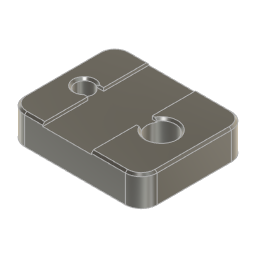
[a]_z_belt_clip_lower_x4 (Autodesk Fusion 360 design; units mm, degrees)
Autodesk Fusion 360 part; units mm, degrees
sketch "Sketch1" plane through (0, 0, 0) normal (0, 0, 1) x (1, 0, 0) in component "Component"
  line L0 (12.5, -10) -> (-12.5, -10)
  line L1 (-12.5, -10) -> (-12.5, 10)
  line L2 (-12.5, 10) -> (12.5, 10)
  line L3 (12.5, 10) -> (12.5, -10)
  line L4 (12.5, -10) -> (-12.5, 10) construction
  line L5 (-12.5, -10) -> (12.5, 10) construction
  line L6 (-12.5, 0) -> (12.5, 0) construction
  line L7 (0, 10) -> (0, -10) construction
  circle A0 centre (-8.25, 0) radius 1.7
  circle A1 centre (6.25, 0) radius 2.7
  dimension "d7" = 25
  dimension "d8" = 20
  dimension "d9" = 3.4
  dimension "d10" = 5.4
  dimension "d11" = 4.25
  dimension "d12" = 6.25
  constraint horizontal L0
  constraint perpendicular L0 L1
  constraint parallel L0 L2
  constraint parallel L1 L3
  constraint coincident L4 origin
  constraint coincident L5 origin
  constraint midpoint L1 L6.start
  constraint midpoint L3 L6.end
  constraint midpoint L2 L7.start
  constraint midpoint L0 L7.end
  constraint coincident L6 A0.centre
  constraint coincident L6 A1.centre
  measures "d7" distance of L1.end L2.end
  measures "d8" distance of L0.end L1.end
  measures "d9" diameter of A0
  measures "d10" diameter of A1
  measures "d11" distance of L1 A0.centre
  measures "d12" distance of L3 A1.centre
extrude "Extrude1" add sketch "Sketch1" along normal mid plane 5.6 in component "Component"
fillet "Fillet1" radius 3 4 edges at (-12.5, -10, 0) (12.5, -10, 0) (12.5, 10, 0) (-12.5, 10, 0) in component "Component"
chamfer "Chamfer1" distance 0.4 angle 45 12 edges at (0, -10, 2.8) (11.6213, -9.1213, 2.8) (12.5, 0, 2.8) (11.6213, 9.1213, 2.8) (0, 10, 2.8) (-11.6213, 9.1213, 2.8) (-12.5, 0, 2.8) (-11.6213, -9.1213, 2.8) (3.7327, 0.9764, 2.8) (-9.835, 0.6147, 2.8) (3.7327, -0.9764, -2.8) (-9.835, -0.6147, -2.8) in component "Component"
sketch "Sketch2" plane through (0, 0, 2.8) normal (0, 0, 1) x (-1, 0, 0) in component "Component"
  circle A0 centre (-6.25, 0) radius 3.1
  line L0 (9.5, 9.6) -> (-9.5, 9.6)
  arc A1 (-9.5, 9.6) -> (-12.1, 7) centre (-9.5, 7) ccw
  line L1 (-12.1, 7) -> (-12.1, -7)
  arc A2 (-12.1, -7) -> (-9.5, -9.6) centre (-9.5, -7) ccw
  line L2 (-9.5, -9.6) -> (9.5, -9.6)
  arc A3 (9.5, -9.6) -> (12.1, -7) centre (9.5, -7) ccw
  line L3 (12.1, -7) -> (12.1, 7)
  arc A4 (12.1, 7) -> (9.5, 9.6) centre (9.5, 7) ccw
  circle A5 centre (8.25, 0) radius 2.1
  line L4 (12.5, -10) -> (-12.5, -10)
  line L5 (12.5, 10) -> (12.5, -10)
  line L6 (-12.5, 10) -> (12.5, 10)
  line L7 (-12.5, -10) -> (-12.5, 10)
  line L8 (6.1, -10) -> (-3.1, -10)
  line L9 (-3.1, -10) -> (-3.1, 10)
  line L10 (-3.1, 10) -> (6.1, 10)
  line L11 (6.1, 10) -> (6.1, -10)
  dimension "d18" = 6.4
  dimension "d19" = 9.4
  constraint horizontal L8
  constraint vertical L9
  constraint horizontal L10
  constraint vertical L11
  constraint coincident L6 L9.end
  constraint coincident L4 L8.start
  measures "d18" distance of L5 L11
  measures "d19" distance of L7 L9
extrude "Extrude2" cut sketch "Sketch2" against normal blind 0.6 contours L0 L2 L9 L11 | L0 L6 L9 L10 L11 | L2 L4 L8 L9 L11 in component "Component"
sketch "Sketch3" plane through (0, 0, 2.8) normal (0, 0, 1) x (-1, 0, 0) in component "Component"
  line L0 (-3.1, -9.6) -> (-3.1, 9.6)
  line L1 (-3.1, 9.6) -> (-9.5, 9.6)
  arc A0 (-9.5, 9.6) -> (-12.1, 7) centre (-9.5, 7) ccw
  line L2 (-12.1, 7) -> (-12.1, -7)
  arc A1 (-12.1, -7) -> (-9.5, -9.6) centre (-9.5, -7) ccw
  line L3 (-9.5, -9.6) -> (-3.1, -9.6)
  circle A2 centre (-6.25, 0) radius 3.1
  line L4 (12.5, -10) -> (-12.5, -10)
  line L5 (12.5, 10) -> (12.5, -10)
  line L6 (-12.5, 10) -> (12.5, 10)
  line L7 (-12.5, -10) -> (-12.5, 10)
  line L8 (-8, 1.5) -> (8, 1.5)
  line L9 (8, 1.5) -> (8, -1.5)
  line L10 (8, -1.5) -> (-8, -1.5)
  line L11 (-8, -1.5) -> (-8, 1.5)
  line L12 (-8, 1.5) -> (8, -1.5) construction
  line L13 (8, 1.5) -> (-8, -1.5) construction
  dimension "d22" = 3
  dimension "d23" = 16
  constraint horizontal L8
  constraint perpendicular L8 L9
  constraint parallel L8 L10
  constraint parallel L9 L11
  constraint coincident L12 origin
  constraint coincident L13 origin
  measures "d22" distance of L8.end L9.end
  measures "d23" distance of L9.end L10.end
extrude "Extrude3" cut sketch "Sketch3" against normal blind 0.6 contours L0 A2 L8 L10 | L0 L8 L9 L10 | A2 L8 L10 L11 picked at (-6.3833, 0) in component "Component"
component "Component" placed x (1, 0, 0) y (0, 1, 0) z (0, 0, 1) at (0, 0, 0)
equation "d13 = ( 5.6 / 2 ) * 1 mm"
